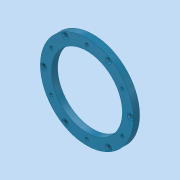
# Autodesk Inventor part: aftSectionAirtightCap
Saved by Autodesk Inventor 2017 (Build 210142000, 142)
## iProperties
Created: 2016-10-25
Part Number: aftSectionAirtightCap
Material: ABS Plastic
Document SubType Name: Modeling
Designer: techn
Density: 1.06 g/cm^3
Appearance: Sky Blue Dark
Mass: 18.7272 g
Surface Area: 100.631 cm^2
Volume: 17.6672 cm^3
Author: techn
Autodesk Inventor part; units mm, degrees
ref_plane "YZ Plane" through (0, 0, 0) normal (1, 0, 0) x (0, 1, 0)
ref_plane "XZ Plane" through (0, 0, 0) normal (0, 1, 0) x (-1, 0, 0)
ref_plane "XY Plane" through (0, 0, 0) normal (0, 0, 1) x (1, 0, 0)
sketch "Sketch1" plane through (0, 0, 0) normal (0, 0, 1) x (1, 0, 0)
  circle A0 centre (0, 0) radius 47.625
  dimension "d0" = 95.25
  constraints: 1 centre point, 1 coincident
  measures "d0" diameter of A0
extrude "Extrusion1" add sketch "Sketch1" along normal blind 6.35
sketch "Sketch2" plane through (0, 0, 6.35) normal (0, 0, 1) x (1, 0, 0)
  circle A0 centre (0, 0) radius 25.4
  dimension "d3" = 50.8
  constraints: 1 centre point, 1 coincident
  measures "d3" diameter of A0
extrude "Extrusion2" cut sketch "Sketch2" against normal blind 6.35
sketch "Sketch3" plane through (0, 0, 6.35) normal (0, 0, 1) x (1, 0, 0)
  line L0 (0, 0) -> (-44.45, 0)
  circle A0 centre (-44.45, 0) radius 1.905
  circle A1 centre (-22.225, -38.4948) radius 1.905
  circle A2 centre (22.225, -38.4948) radius 1.905
  circle A3 centre (44.45, 0) radius 1.905
  circle A4 centre (22.225, 38.4948) radius 1.905
  circle A5 centre (-22.225, 38.4948) radius 1.905
  dimension "d6" = 3.81
  dimension "d7" = 44.45
  dimension "d10" = 360
  constraints: 6 centre point, 2 end point, 1 coincident, 1 horizontal, 13 other
  measures "d6" diameter of A0
  measures "d7" distance of L0.start L0.end
extrude "Extrusion3" cut sketch "Sketch3" against normal blind 6.35
chamfer "Chamfer1" distance 1.27 angle 45 6 edges at (-24.13, 38.4948, 6.35) (-46.355, 0, 6.35) (-24.13, -38.4948, 6.35) (20.32, 38.4948, 6.35) (42.545, 0, 6.35) (20.32, -38.4948, 6.35)
sketch "Sketch4" plane through (0, 0, 6.35) normal (0, 0, 1) x (1, 0, 0)
  circle A0 centre (0, 41.91) radius 1.5875
  circle A1 centre (-36.2951, 20.955) radius 1.5875
  circle A2 centre (-36.2951, -20.955) radius 1.5875
  circle A3 centre (0, -41.91) radius 1.5875
  circle A4 centre (36.2951, -20.955) radius 1.5875
  circle A5 centre (36.2951, 20.955) radius 1.5875
  point P0 (0, 0)
  dimension "d17" = 3.175
  dimension "d18" = 41.91
  dimension "d21" = 360
  constraints: 6 centre point, 13 other
  measures "d17" diameter of A0
  measures "d18" distance of A0.centre point (0, 0)
extrude "Extrusion4" cut sketch "Sketch4" against normal blind 25.4
sketch "Sketch5" plane through (0, 0, 0) normal (0, 0, -1) x (-1, 0, 0)
  circle A0 centre (0, 41.91) radius 1.5875 projected
  line L0 (-3.8861, 41.91) -> (-1.9431, 45.2755)
  line L1 (-1.9431, 45.2755) -> (1.9431, 45.2755)
  line L2 (1.9431, 45.2755) -> (3.8861, 41.91)
  line L3 (3.8861, 41.91) -> (1.9431, 38.5445)
  line L4 (1.9431, 38.5445) -> (-1.9431, 38.5445)
  line L5 (-1.9431, 38.5445) -> (-3.8861, 41.91)
  line L6 (-38.2382, 17.5895) -> (-40.1813, 20.955)
  line L7 (-40.1813, 20.955) -> (-38.2382, 24.3205)
  line L8 (-38.2382, 24.3205) -> (-34.3521, 24.3205)
  line L9 (-34.3521, 24.3205) -> (-32.409, 20.955)
  line L10 (-32.409, 20.955) -> (-34.3521, 17.5895)
  line L11 (-34.3521, 17.5895) -> (-38.2382, 17.5895)
  line L12 (-34.3521, -24.3205) -> (-38.2382, -24.3205)
  line L13 (-38.2382, -24.3205) -> (-40.1813, -20.955)
  line L14 (-40.1813, -20.955) -> (-38.2382, -17.5895)
  line L15 (-38.2382, -17.5895) -> (-34.3521, -17.5895)
  line L16 (-34.3521, -17.5895) -> (-32.409, -20.955)
  line L17 (-32.409, -20.955) -> (-34.3521, -24.3205)
  line L18 (3.8861, -41.91) -> (1.9431, -45.2755)
  line L19 (1.9431, -45.2755) -> (-1.9431, -45.2755)
  line L20 (-1.9431, -45.2755) -> (-3.8861, -41.91)
  line L21 (-3.8861, -41.91) -> (-1.9431, -38.5445)
  line L22 (-1.9431, -38.5445) -> (1.9431, -38.5445)
  line L23 (1.9431, -38.5445) -> (3.8861, -41.91)
  line L24 (38.2382, -17.5895) -> (40.1813, -20.955)
  line L25 (40.1813, -20.955) -> (38.2382, -24.3205)
  line L26 (38.2382, -24.3205) -> (34.3521, -24.3205)
  line L27 (34.3521, -24.3205) -> (32.409, -20.955)
  line L28 (32.409, -20.955) -> (34.3521, -17.5895)
  line L29 (34.3521, -17.5895) -> (38.2382, -17.5895)
  line L30 (34.3521, 24.3205) -> (38.2382, 24.3205)
  line L31 (38.2382, 24.3205) -> (40.1813, 20.955)
  line L32 (40.1813, 20.955) -> (38.2382, 17.5895)
  line L33 (38.2382, 17.5895) -> (34.3521, 17.5895)
  line L34 (34.3521, 17.5895) -> (32.409, 20.955)
  line L35 (32.409, 20.955) -> (34.3521, 24.3205)
  point P0 (0, 0)
  point P1 (-36.2951, 20.955)
  point P2 (-36.2951, -20.955)
  point P3 (0, -41.91)
  point P4 (36.2951, -20.955)
  point P5 (36.2951, 20.955)
  dimension "d25" = 6.731
  dimension "d28" = 360
  constraints: 72 end point, 1 coincident, 92 other
  measures "d25" distance between parallel lines of L1 L4
extrude "Extrusion5" cut sketch "Sketch5" against normal blind 2.3813
sketch "Sketch6" plane through (0, 0, 6.35) normal (0, 0, 1) x (1, 0, 0)
  circle A0 centre (20.795, 25.8191) radius 3.175
  line L0 (0, 0) -> (0, 9.7848)
  circle A1 centre (-20.795, 25.8191) radius 3.175
  dimension "d32" = 6.35
  dimension "d33" = 20.795
  dimension "d34" = 25.8191
  constraints: 2 centre point, 2 end point, 1 symmetric about line, 1 vertical, 1 other
  measures "d32" diameter of A0
  measures "d33" horizontal distance of A0.centre L0.start
  measures "d34" vertical distance of A0.centre L0.start
extrude "Extrusion6" cut sketch "Sketch6" against normal blind 25.4
sketch "Sketch7" plane through (0, 0, 0) normal (0, 0, -1) x (-1, 0, 0)
  circle A0 centre (-20.795, 25.8191) radius 3.175 projected
  circle A1 centre (20.795, 25.8191) radius 3.175 projected
  line L0 (32.409, 20.955) -> (34.3521, 24.3205) projected
  line L1 (34.3521, 24.3205) -> (38.2382, 24.3205) projected
  line L2 (38.2382, 24.3205) -> (40.1813, 20.955) projected
  line L3 (40.1813, 20.955) -> (38.2382, 17.5895) projected
  line L4 (38.2382, 17.5895) -> (34.3521, 17.5895) projected
  line L5 (34.3521, 17.5895) -> (32.409, 20.955) projected
  line L6 (1.9431, -38.5445) -> (3.8861, -41.91) projected
  line L7 (3.8861, -41.91) -> (1.9431, -45.2755) projected
  line L8 (1.9431, -45.2755) -> (-1.9431, -45.2755) projected
  line L9 (-1.9431, -45.2755) -> (-3.8861, -41.91) projected
  line L10 (-3.8861, -41.91) -> (-1.9431, -38.5445) projected
  line L11 (-1.9431, -38.5445) -> (1.9431, -38.5445) projected
  line L12 (-34.3521, 17.5895) -> (-38.2382, 17.5895) projected
  line L13 (-38.2382, 17.5895) -> (-40.1813, 20.955) projected
  line L14 (-40.1813, 20.955) -> (-38.2382, 24.3205) projected
  line L15 (-38.2382, 24.3205) -> (-34.3521, 24.3205) projected
  line L16 (-34.3521, 24.3205) -> (-32.409, 20.955) projected
  line L17 (-32.409, 20.955) -> (-34.3521, 17.5895) projected
  line L18 (-1.9431, 38.5445) -> (-3.8861, 41.91) projected
  line L19 (-3.8861, 41.91) -> (-1.9431, 45.2755) projected
  line L20 (-1.9431, 45.2755) -> (1.9431, 45.2755) projected
  line L21 (1.9431, 45.2755) -> (3.8861, 41.91) projected
  line L22 (3.8861, 41.91) -> (1.9431, 38.5445) projected
  line L23 (1.9431, 38.5445) -> (-1.9431, 38.5445) projected
  line L24 (-32.409, -20.955) -> (-34.3521, -24.3205) projected
  line L25 (-34.3521, -24.3205) -> (-38.2382, -24.3205) projected
  line L26 (-38.2382, -24.3205) -> (-40.1813, -20.955) projected
  line L27 (-40.1813, -20.955) -> (-38.2382, -17.5895) projected
  line L28 (-38.2382, -17.5895) -> (-34.3521, -17.5895) projected
  line L29 (-34.3521, -17.5895) -> (-32.409, -20.955) projected
  line L30 (34.3521, -17.5895) -> (38.2382, -17.5895) projected
  line L31 (38.2382, -17.5895) -> (40.1813, -20.955) projected
  line L32 (40.1813, -20.955) -> (38.2382, -24.3205) projected
  line L33 (38.2382, -24.3205) -> (34.3521, -24.3205) projected
  line L34 (34.3521, -24.3205) -> (32.409, -20.955) projected
  line L35 (32.409, -20.955) -> (34.3521, -17.5895) projected
  circle A2 centre (-22.225, 38.4948) radius 1.905 projected
  circle A3 centre (-22.225, -38.4948) radius 1.905 projected
  circle A4 centre (44.45, 0) radius 1.905 projected
  circle A5 centre (22.225, -38.4948) radius 1.905 projected
  circle A6 centre (-44.45, 0) radius 1.905 projected
  circle A7 centre (22.225, 38.4948) radius 1.905 projected
  circle A8 centre (0, 0) radius 25.4 projected
  circle A9 centre (0, 0) radius 47.625 projected
  circle A10 centre (0, 0) radius 36.327
  constraints: 1 centre point, 1 coincident, 1 tangent
extrude "Extrusion7" cut sketch "Sketch7" against normal blind 25.4 contours A10
body "Solid1"
